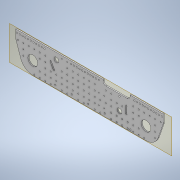
# Autodesk Inventor part: inside_plate
Saved by Autodesk Inventor 2022 (Build 260153000, 153)
## iProperties
Created: 2021-07-14
Part Number: inside_plate
Material: Generic
Document SubType Name: Modeling
Designer: gfellows
Density: 1 g/cm^3
Appearance: Default
Author: gfellows
Autodesk Inventor part; units mm, degrees
ref_plane "YZ Plane" through (0, 0, 0) normal (1, 0, 0) x (0, 1, 0)
ref_plane "XZ Plane" through (0, 0, 0) normal (0, 1, 0) x (-1, 0, 0)
ref_plane "XY Plane" through (0, 0, 0) normal (0, 0, 1) x (1, 0, 0)
ref_plane "Work Plane1" through (165.1, 7.35, 75.175) normal (0, 0, 1) x (1, 0, 0)
sketch "Sketch1" plane through (165.1, 7.35, 75.175) normal (0, 0, 1) x (1, 0, 0)
  circle A0 centre (165.1, -7.35) radius 14.2748 projected
  circle A1 centre (-165.1, -7.35) radius 14.2748 projected
  circle A2 centre (87.5579, -8.15) radius 7.008 projected
  circle A3 centre (-97.8958, 31.6508) radius 7.008 construction
  line L0 (59.5579, -27.1492) -> (-64.3191, -27.1492) construction
  line L1 (-64.3191, 10.8492) -> (59.5579, 10.8492) construction
  line L2 (-64.3191, -27.1492) -> (-64.3191, 10.8492) construction
  line L3 (59.5579, 10.8492) -> (59.5579, -27.1492) construction
  line L4 (73.4511, 1.35) -> (73.4511, -17.65) construction
  line L5 (59.5579, 1.35) -> (73.4511, 1.35) construction
  line L6 (73.4511, -17.65) -> (59.5579, -17.65) construction
  line L7 (113.5579, -44.65) -> (89.5579, -44.65) construction
  line L8 (89.5579, -44.65) -> (89.5579, -20.65) construction
  line L9 (85.5579, -20.65) -> (85.5579, -44.65) construction
  line L10 (85.5579, -44.65) -> (61.5579, -44.65) construction
  line L11 (61.5579, -44.65) -> (61.5579, -20.65) construction
  line L12 (61.5579, -20.65) -> (85.5579, -20.65) construction
  line L13 (89.5579, -20.65) -> (113.5579, -20.65) construction
  line L14 (113.5579, -20.65) -> (113.5579, -44.65) construction
  arc A4 (56.5579, -44.65) -> (60.5579, -40.65) centre (56.5579, -40.65) ccw construction
  arc A5 (-200.3988, -19.4033) -> (-165.1, -44.65) centre (-165.1, -7.35) ccw projected
  line L15 (215.1, 47.65) -> (-215.1, 47.65) projected
  arc A6 (165.1, -44.65) -> (200.3988, -19.4033) centre (165.1, -7.35) ccw projected
  arc A7 (114.5579, -40.65) -> (118.5579, -44.65) centre (118.5579, -40.65) ccw construction
  line L16 (114.5579, -23.65) -> (114.5579, -40.65) construction
  arc A8 (114.5579, -23.65) -> (110.5579, -19.65) centre (110.5579, -23.65) ccw construction
  line L17 (64.5579, -19.65) -> (110.5579, -19.65) construction
  arc A9 (64.5579, -19.65) -> (60.5579, -23.65) centre (64.5579, -23.65) ccw construction
  line L18 (60.5579, -40.65) -> (60.5579, -23.65) construction
  circle A10 centre (-165.1, -7.35) radius 14.2748 projected
  circle A11 centre (165.1, -7.35) radius 14.2748 projected
  circle A12 centre (-96.2421, 28.6508) radius 7.008 projected
  circle A13 centre (87.5579, -8.15) radius 7.008 projected
  line L19 (56.5579, -44.65) -> (118.5579, -44.65)
  circle A14 centre (63.5579, -24.65) radius 2
  circle A15 centre (79.5579, -24.65) radius 2
  circle A16 centre (63.5579, -40.65) radius 2
  circle A17 centre (79.5579, -40.65) radius 2
  circle A18 centre (95.5579, -24.65) radius 2
  circle A19 centre (111.5579, -24.65) radius 2
  circle A20 centre (111.5579, -40.65) radius 2
  circle A21 centre (95.5579, -40.65) radius 2
  circle A22 centre (27.1704, 7.85) radius 1.3526
  circle A23 centre (43.1704, 7.85) radius 1.3526
  circle A24 centre (27.1704, -24.15) radius 1.3526
  circle A25 centre (43.1704, -24.15) radius 1.3526
  line L20 (27.1704, 7.85) -> (43.1704, -24.15) construction
  line L21 (73.4511, -8.15) -> (-64.3191, -8.15) construction
  line L22 (-165.1, -44.65) -> (56.5579, -44.65) projected
  line L23 (-214.6708, 22.3931) -> (-200.3988, -19.4033) projected
  line L24 (-215.1, 47.65) -> (-215.1, 24.9782) projected
  line L25 (200.3988, -19.4033) -> (214.6708, 22.3931) projected
  line L26 (118.5579, -44.65) -> (165.1, -44.65) projected
  arc A26 (214.6708, 22.3931) -> (215.1, 24.9782) centre (207.1, 24.9782) ccw projected
  arc A27 (-215.1, 24.9782) -> (-214.6708, 22.3931) centre (-207.1, 24.9782) ccw projected
  circle A28 centre (-4.9, 39.65) radius 2 projected
  line L27 (31.1, 47.65) -> (31.1, 35.65) projected
  line L28 (-56.9, 47.65) -> (31.1, 47.65) projected
  line L29 (-56.9, 47.65) -> (-56.9, 35.65) projected
  line L30 (-56.9, 35.65) -> (31.1, 35.65) projected
  circle A29 centre (11.1, 39.65) radius 2 projected
  circle A30 centre (3.1, 39.65) radius 2 projected
  circle A31 centre (-4.9, 39.65) radius 2 projected
  circle A32 centre (-12.9, 39.65) radius 2 projected
  circle A33 centre (-20.9, 39.65) radius 2 projected
  circle A34 centre (-28.9, 39.65) radius 2 projected
  circle A35 centre (-36.9, 39.65) radius 2 projected
  circle A36 centre (-44.9, 39.65) radius 2 projected
  circle A37 centre (-52.9, 39.65) radius 2 projected
  circle A38 centre (19.1, 39.65) radius 2 projected
  circle A39 centre (27.1, 39.65) radius 2 projected
  line L31 (-215.1, 45.15) -> (-127.1, 45.15) projected
  line L32 (-127.1, 47.65) -> (-127.1, 35.65) projected
  line L33 (-215.1, 47.65) -> (-127.1, 47.65) projected
  line L34 (-215.1, 47.65) -> (-215.1, 35.65) projected
  line L35 (-215.1, 35.65) -> (-127.1, 35.65) projected
  circle A40 centre (-147.1, 39.65) radius 2 projected
  circle A41 centre (-155.1, 39.65) radius 2 projected
  circle A42 centre (-163.1, 39.65) radius 2 projected
  circle A43 centre (-171.1, 39.65) radius 2 projected
  circle A44 centre (-179.1, 39.65) radius 2 projected
  circle A45 centre (-187.1, 39.65) radius 2 projected
  circle A46 centre (-195.1, 39.65) radius 2 projected
  circle A47 centre (-203.1, 39.65) radius 2 projected
  circle A48 centre (-211.1, 39.65) radius 2 projected
  circle A49 centre (-139.1, 39.65) radius 2 projected
  circle A50 centre (-131.1, 39.65) radius 2 projected
  line L36 (215.1, 47.65) -> (215.1, 35.65) projected
  line L37 (127.1, 47.65) -> (215.1, 47.65) projected
  line L38 (127.1, 47.65) -> (127.1, 35.65) projected
  line L39 (127.1, 35.65) -> (215.1, 35.65) projected
  circle A51 centre (195.1, 39.65) radius 2 projected
  circle A52 centre (187.1, 39.65) radius 2 projected
  circle A53 centre (179.1, 39.65) radius 2 projected
  circle A54 centre (171.1, 39.65) radius 2 projected
  circle A55 centre (163.1, 39.65) radius 2 projected
  circle A56 centre (155.1, 39.65) radius 2 projected
  circle A57 centre (147.1, 39.65) radius 2 projected
  circle A58 centre (139.1, 39.65) radius 2 projected
  circle A59 centre (131.1, 39.65) radius 2 projected
  circle A60 centre (203.1, 39.65) radius 2 projected
  circle A61 centre (211.1, 39.65) radius 2 projected
  line L40 (215.1, 24.9782) -> (215.1, 47.65) projected
  arc A62 (109.4269, 14.5493) -> (105.4269, 14.5493) centre (107.4269, 14.5493) ccw projected
  line L41 (105.4269, -5.4507) -> (105.4269, 14.5493) projected
  arc A63 (105.4269, -5.4507) -> (109.4269, -5.4507) centre (107.4269, -5.4507) ccw projected
  line L42 (109.4269, 14.5493) -> (109.4269, -5.4507) projected
  arc A64 (-105.2208, -1.6588) -> (-101.6761, 0.1945) centre (-103.4484, -0.7322) ccw projected
  line L43 (-110.9425, 17.9183) -> (-101.6761, 0.1945) projected
  arc A65 (-110.9425, 17.9183) -> (-114.4873, 16.065) centre (-112.7149, 16.9916) ccw projected
  line L44 (-105.2208, -1.6588) -> (-114.4873, 16.065) projected
  circle A66 centre (-139.1, 39.65) radius 2 projected
  circle A67 centre (-155.1, 39.65) radius 2 projected
  circle A68 centre (-179.1, 39.65) radius 2 projected
  circle A69 centre (-187.1, 39.65) radius 2 projected
  circle A70 centre (-203.1, 39.65) radius 2 projected
  circle A71 centre (211.1, 39.65) radius 2 projected
  circle A72 centre (195.1, 39.65) radius 2 projected
  circle A73 centre (179.1, 39.65) radius 2 projected
  circle A74 centre (163.1, 39.65) radius 2 projected
  circle A75 centre (131.1, 39.65) radius 2 projected
  circle A76 centre (139.1, 39.65) radius 2 projected
  circle A77 centre (147.1, 39.65) radius 2 projected
  circle A78 centre (155.1, 39.65) radius 2 projected
  circle A79 centre (171.1, 39.65) radius 2 projected
  circle A80 centre (187.1, 39.65) radius 2 projected
  circle A81 centre (203.1, 39.65) radius 2 projected
  circle A82 centre (-211.1, 39.65) radius 2 projected
  circle A83 centre (-195.1, 39.65) radius 2 projected
  circle A84 centre (-171.1, 39.65) radius 2 projected
  circle A85 centre (-163.1, 39.65) radius 2 projected
  circle A86 centre (-147.1, 39.65) radius 2 projected
  circle A87 centre (-131.1, 39.65) radius 2 projected
  circle A88 centre (87.5579, 28.6508) radius 2 projected
  circle A89 centre (-99.4421, -35.8996) radius 2 projected
  circle A90 centre (-51.4421, -35.8996) radius 2 projected
  circle A91 centre (-3.4421, -35.8996) radius 2 projected
  circle A92 centre (44.5579, -35.8996) radius 2 projected
  circle A93 centre (119.5579, -39.65) radius 2 projected
  line L45 (63.5579, -24.65) -> (79.5579, -40.65) construction
  line L46 (95.5579, -24.65) -> (111.5579, -40.65) construction
  line L47 (63.5579, -40.65) -> (79.5579, -24.65) construction
  line L48 (95.5579, -40.65) -> (111.5579, -24.65) construction
  circle A94 centre (-96.2421, 28.6508) radius 6.25 construction
  circle A95 centre (-96.2421, 28.6508) radius 13.4851 projected
  circle A96 centre (-97.8958, 31.6508) radius 6.35 construction
  circle A97 centre (-96.2421, 28.6508) radius 7.0079
  circle A98 centre (52.9299, -33.2) radius 1.65 projected
  circle A99 centre (52.9299, 43) radius 1.65 projected
  circle A100 centre (-124.8701, -33.2) radius 1.65 projected
  circle A101 centre (-124.8701, 43) radius 1.65 projected
  point P0 (35.1704, -8.15)
  point P1 (207.1, 24.9782)
  point P2 (71.5579, -32.65)
  point P3 (103.5579, -32.65)
  dimension "d2" = 4
  dimension "d5" = 16
  dimension "d8" = 16
  dimension "d11" = 4
  dimension "d12" = 2
  dimension "d15" = 32
  dimension "d20" = 2.7051
  dimension "d23" = 16
  dimension "d30" = 31.9999
  dimension "d35" = 52.3875
  dimension "d36" = 32
  dimension "d37" = 12.7
  dimension "d38" = 14.0157
  constraints: 14 centre point, 14 end point, 5 midpoint, 4 horizontal, 2 coincident, 2 vertical, 1 point on line, 1 tangent, 20 other
  measures "d2" diameter of A14
  measures "d5" distance of L45.start L47.end
  measures "d8" distance of L45.start L47.start
  measures "d11" distance from line of L12 L45.start
  measures "d12" distance from line of L11 L45.start
  measures "d15" distance of L45.start L46.start
  measures "d20" diameter of A22
  measures "d23" distance of L20.start A23.centre
  measures "d30" distance of L20.start A24.centre
  measures "d35" distance of A2.centre point (35.17, -8.15)
  measures "d36" distance of point (103.558, -32.65) point (71.558, -32.65)
  measures "d37" diameter of A96
  measures "d38" diameter of A97
extrude "Extrusion1" add sketch "Sketch1" along normal blind 3.175 contours L23 A27 L24 L35 L32 L15 L29 L30 L27 L38 L39 L40 A26 L25 A6 L26 L19 L22 A5 | L24 L31 L32 L35 | L24 L15 L32 L31 | L15 L27 L30 L29 | L39 L38 L15 L36 | A95 | A98 | A99 | A100 | A101
sketch "Sketch2" plane through (165.1, 7.35, 78.35) normal (0, 0, 1) x (1, 0, 0)
  circle A0 centre (63.5579, -24.65) radius 2 projected
  circle A1 centre (79.5579, -24.65) radius 2 projected
  circle A2 centre (79.5579, -40.65) radius 2 projected
  circle A3 centre (63.5579, -40.65) radius 2 projected
  line L0 (215.1, 24.9782) -> (215.1, 47.65) projected
  line L1 (215.1, 47.65) -> (-215.1, 47.65) projected
  line L2 (-215.1, 47.65) -> (-215.1, 24.9782) projected
  arc A4 (-215.1, 24.9782) -> (-214.6708, 22.3931) centre (-207.1, 24.9782) ccw projected
  line L3 (-214.6708, 22.3931) -> (-200.3988, -19.4033) projected
  arc A5 (-200.3988, -19.4033) -> (-165.1, -44.65) centre (-165.1, -7.35) ccw projected
  line L4 (-165.1, -44.65) -> (165.1, -44.65) projected
  arc A6 (165.1, -44.65) -> (200.3988, -19.4033) centre (165.1, -7.35) ccw projected
  line L5 (200.3988, -19.4033) -> (214.6708, 22.3931) projected
  arc A7 (214.6708, 22.3931) -> (215.1, 24.9782) centre (207.1, 24.9782) ccw projected
  circle A8 centre (-131.1, 39.65) radius 2 projected
  circle A9 centre (-211.1, 39.65) radius 2 projected
  circle A10 centre (-147.1, 39.65) radius 2 projected
  circle A11 centre (-155.1, 39.65) radius 2 projected
  circle A12 centre (-163.1, 39.65) radius 2 projected
  circle A13 centre (-171.1, 39.65) radius 2 projected
  circle A14 centre (-179.1, 39.65) radius 2 projected
  circle A15 centre (-187.1, 39.65) radius 2 projected
  circle A16 centre (-195.1, 39.65) radius 2 projected
  circle A17 centre (-203.1, 39.65) radius 2 projected
  circle A18 centre (-139.1, 39.65) radius 2 projected
  circle A19 centre (211.1, 39.65) radius 2 projected
  circle A20 centre (131.1, 39.65) radius 2 projected
  circle A21 centre (195.1, 39.65) radius 2 projected
  circle A22 centre (187.1, 39.65) radius 2 projected
  circle A23 centre (179.1, 39.65) radius 2 projected
  circle A24 centre (171.1, 39.65) radius 2 projected
  circle A25 centre (163.1, 39.65) radius 2 projected
  circle A26 centre (155.1, 39.65) radius 2 projected
  circle A27 centre (147.1, 39.65) radius 2 projected
  circle A28 centre (139.1, 39.65) radius 2 projected
  circle A29 centre (203.1, 39.65) radius 2 projected
  circle A30 centre (27.1, 39.65) radius 2 projected
  circle A31 centre (-52.9, 39.65) radius 2 projected
  circle A32 centre (-36.9, 39.65) radius 2 projected
  circle A33 centre (-20.9, 39.65) radius 2 projected
  circle A34 centre (3.1, 39.65) radius 2 projected
  circle A35 centre (-4.9, 39.65) radius 2 projected
  circle A36 centre (11.1, 39.65) radius 2 projected
  circle A37 centre (-12.9, 39.65) radius 2 projected
  circle A38 centre (-28.9, 39.65) radius 2 projected
  circle A39 centre (-44.9, 39.65) radius 2 projected
  circle A40 centre (19.1, 39.65) radius 2 projected
  circle A41 centre (-96.2421, 28.6508) radius 7.0079 projected
  line L6 (105.4269, -5.4507) -> (105.4269, 14.5493) projected
  arc A42 (109.4269, 14.5493) -> (105.4269, 14.5493) centre (107.4269, 14.5493) ccw projected
  line L7 (109.4269, 14.5493) -> (109.4269, -5.4507) projected
  arc A43 (105.4269, -5.4507) -> (109.4269, -5.4507) centre (107.4269, -5.4507) ccw projected
  line L8 (-110.9425, 17.9183) -> (-101.6761, 0.1945) projected
  arc A44 (-105.2208, -1.6588) -> (-101.6761, 0.1945) centre (-103.4484, -0.7322) ccw projected
  line L9 (-105.2208, -1.6588) -> (-114.4873, 16.065) projected
  arc A45 (-110.9425, 17.9183) -> (-114.4873, 16.065) centre (-112.7149, 16.9916) ccw projected
  circle A46 centre (44.5579, -35.8996) radius 2 projected
  circle A47 centre (-51.4421, -35.8996) radius 2 projected
  circle A48 centre (87.5579, 28.6508) radius 2 projected
  circle A49 centre (27.1704, -24.15) radius 1.3526 projected
  circle A50 centre (27.1704, 7.85) radius 1.3526 projected
  circle A51 centre (111.5579, -40.65) radius 2 projected
  circle A52 centre (95.5579, -24.65) radius 2 projected
  circle A53 centre (165.1, -7.35) radius 14.2748 projected
  circle A54 centre (-165.1, -7.35) radius 14.2748 projected
  circle A55 centre (87.5579, -8.15) radius 7.008 projected
  circle A56 centre (63.5579, -24.65) radius 2 projected
  circle A57 centre (79.5579, -24.65) radius 2 projected
  circle A58 centre (63.5579, -40.65) radius 2 projected
  circle A59 centre (79.5579, -40.65) radius 2 projected
  circle A60 centre (111.5579, -24.65) radius 2 projected
  circle A61 centre (95.5579, -40.65) radius 2 projected
  circle A62 centre (43.1704, 7.85) radius 1.3526 projected
  circle A63 centre (43.1704, -24.15) radius 1.3526 projected
  circle A64 centre (-99.4421, -35.8996) radius 2 projected
  circle A65 centre (-3.4421, -35.8996) radius 2 projected
  circle A66 centre (119.5579, -39.65) radius 2 projected
  circle A67 centre (-203.1, 39.65) radius 1.65
  circle A68 centre (111.5579, -40.65) radius 2 projected
  circle A69 centre (111.5579, -40.65) radius 1.65
  circle A70 centre (95.5579, -40.65) radius 1.65
  circle A71 centre (79.5579, -40.65) radius 1.65
  circle A72 centre (63.5579, -40.65) radius 1.65
  circle A73 centre (47.5579, -40.65) radius 1.65
  circle A74 centre (31.5579, -40.65) radius 1.65
  circle A75 centre (15.5579, -40.65) radius 1.65
  circle A76 centre (-0.4421, -40.65) radius 1.65
  circle A77 centre (-16.4421, -40.65) radius 1.65
  circle A78 centre (-32.4421, -40.65) radius 1.65
  circle A79 centre (-48.4421, -40.65) radius 1.65
  circle A80 centre (-64.4421, -40.65) radius 1.65
  circle A81 centre (-80.4421, -40.65) radius 1.65
  circle A82 centre (-96.4421, -40.65) radius 1.65
  circle A83 centre (-112.4421, -40.65) radius 1.65
  circle A84 centre (-128.4421, -40.65) radius 1.65
  circle A85 centre (-144.4421, -40.65) radius 1.65
  circle A86 centre (-160.4421, -40.65) radius 1.65
  circle A87 centre (-176.4421, -40.65) radius 1.65
  circle A88 centre (-192.4421, -40.65) radius 1.65
  circle A89 centre (-208.4421, -40.65) radius 1.65
  circle A90 centre (111.5579, -24.65) radius 1.65
  circle A91 centre (95.5579, -24.65) radius 1.65
  circle A92 centre (79.5579, -24.65) radius 1.65
  circle A93 centre (63.5579, -24.65) radius 1.65
  circle A94 centre (47.5579, -24.65) radius 1.65
  circle A95 centre (31.5579, -24.65) radius 1.65
  circle A96 centre (15.5579, -24.65) radius 1.65
  circle A97 centre (-0.4421, -24.65) radius 1.65
  circle A98 centre (-16.4421, -24.65) radius 1.65
  circle A99 centre (-32.4421, -24.65) radius 1.65
  circle A100 centre (-48.4421, -24.65) radius 1.65
  circle A101 centre (-64.4421, -24.65) radius 1.65
  circle A102 centre (-80.4421, -24.65) radius 1.65
  circle A103 centre (-96.4421, -24.65) radius 1.65
  circle A104 centre (-112.4421, -24.65) radius 1.65
  circle A105 centre (-128.4421, -24.65) radius 1.65
  circle A106 centre (-144.4421, -24.65) radius 1.65
  circle A107 centre (-160.4421, -24.65) radius 1.65
  circle A108 centre (-176.4421, -24.65) radius 1.65
  circle A109 centre (-192.4421, -24.65) radius 1.65
  circle A110 centre (-208.4421, -24.65) radius 1.65
  circle A111 centre (111.5579, -8.65) radius 1.65
  circle A112 centre (95.5579, -8.65) radius 1.65
  circle A113 centre (79.5579, -8.65) radius 1.65
  circle A114 centre (63.5579, -8.65) radius 1.65
  circle A115 centre (47.5579, -8.65) radius 1.65
  circle A116 centre (31.5579, -8.65) radius 1.65
  circle A117 centre (15.5579, -8.65) radius 1.65
  circle A118 centre (-0.4421, -8.65) radius 1.65
  circle A119 centre (-16.4421, -8.65) radius 1.65
  circle A120 centre (-32.4421, -8.65) radius 1.65
  circle A121 centre (-48.4421, -8.65) radius 1.65
  circle A122 centre (-64.4421, -8.65) radius 1.65
  circle A123 centre (-80.4421, -8.65) radius 1.65
  circle A124 centre (-96.4421, -8.65) radius 1.65
  circle A125 centre (-112.4421, -8.65) radius 1.65
  circle A126 centre (-128.4421, -8.65) radius 1.65
  circle A127 centre (-144.4421, -8.65) radius 1.65
  circle A128 centre (-160.4421, -8.65) radius 1.65
  circle A129 centre (-176.4421, -8.65) radius 1.65
  circle A130 centre (-192.4421, -8.65) radius 1.65
  circle A131 centre (-208.4421, -8.65) radius 1.65
  circle A132 centre (111.5579, 7.35) radius 1.65
  circle A133 centre (95.5579, 7.35) radius 1.65
  circle A134 centre (79.5579, 7.35) radius 1.65
  circle A135 centre (63.5579, 7.35) radius 1.65
  circle A136 centre (47.5579, 7.35) radius 1.65
  circle A137 centre (31.5579, 7.35) radius 1.65
  circle A138 centre (15.5579, 7.35) radius 1.65
  circle A139 centre (-0.4421, 7.35) radius 1.65
  circle A140 centre (-16.4421, 7.35) radius 1.65
  circle A141 centre (-32.4421, 7.35) radius 1.65
  circle A142 centre (-48.4421, 7.35) radius 1.65
  circle A143 centre (-64.4421, 7.35) radius 1.65
  circle A144 centre (-80.4421, 7.35) radius 1.65
  circle A145 centre (-96.4421, 7.35) radius 1.65
  circle A146 centre (-112.4421, 7.35) radius 1.65
  circle A147 centre (-128.4421, 7.35) radius 1.65
  circle A148 centre (-144.4421, 7.35) radius 1.65
  circle A149 centre (-160.4421, 7.35) radius 1.65
  circle A150 centre (-176.4421, 7.35) radius 1.65
  circle A151 centre (-192.4421, 7.35) radius 1.65
  circle A152 centre (-208.4421, 7.35) radius 1.65
  circle A153 centre (111.5579, 23.35) radius 1.65
  circle A154 centre (95.5579, 23.35) radius 1.65
  circle A155 centre (79.5579, 23.35) radius 1.65
  circle A156 centre (63.5579, 23.35) radius 1.65
  circle A157 centre (47.5579, 23.35) radius 1.65
  circle A158 centre (31.5579, 23.35) radius 1.65
  circle A159 centre (15.5579, 23.35) radius 1.65
  circle A160 centre (-0.4421, 23.35) radius 1.65
  circle A161 centre (-16.4421, 23.35) radius 1.65
  circle A162 centre (-32.4421, 23.35) radius 1.65
  circle A163 centre (-48.4421, 23.35) radius 1.65
  circle A164 centre (-64.4421, 23.35) radius 1.65
  circle A165 centre (-80.4421, 23.35) radius 1.65
  circle A166 centre (-96.4421, 23.35) radius 1.65
  circle A167 centre (-112.4421, 23.35) radius 1.65
  circle A168 centre (-128.4421, 23.35) radius 1.65
  circle A169 centre (-144.4421, 23.35) radius 1.65
  circle A170 centre (-160.4421, 23.35) radius 1.65
  circle A171 centre (-176.4421, 23.35) radius 1.65
  circle A172 centre (-192.4421, 23.35) radius 1.65
  circle A173 centre (-208.4421, 23.35) radius 1.65
  circle A174 centre (111.5579, 39.35) radius 1.65
  circle A175 centre (95.5579, 39.35) radius 1.65
  circle A176 centre (79.5579, 39.35) radius 1.65
  circle A177 centre (63.5579, 39.35) radius 1.65
  circle A178 centre (47.5579, 39.35) radius 1.65
  circle A179 centre (31.5579, 39.35) radius 1.65
  circle A180 centre (15.5579, 39.35) radius 1.65
  circle A181 centre (-0.4421, 39.35) radius 1.65
  circle A182 centre (-16.4421, 39.35) radius 1.65
  circle A183 centre (-32.4421, 39.35) radius 1.65
  circle A184 centre (-48.4421, 39.35) radius 1.65
  circle A185 centre (-64.4421, 39.35) radius 1.65
  circle A186 centre (-80.4421, 39.35) radius 1.65
  circle A187 centre (-96.4421, 39.35) radius 1.65
  circle A188 centre (-112.4421, 39.35) radius 1.65
  circle A189 centre (-128.4421, 39.35) radius 1.65
  circle A190 centre (-144.4421, 39.35) radius 1.65
  circle A191 centre (-160.4421, 39.35) radius 1.65
  circle A192 centre (-176.4421, 39.35) radius 1.65
  circle A193 centre (-192.4421, 39.35) radius 1.65
  circle A194 centre (-208.4421, 39.35) radius 1.65
  circle A195 centre (127.5579, -40.65) radius 1.65
  circle A196 centre (143.5579, -40.65) radius 1.65
  circle A197 centre (159.5579, -40.65) radius 1.65
  circle A198 centre (175.5579, -40.65) radius 1.65
  circle A199 centre (191.5579, -40.65) radius 1.65
  circle A200 centre (207.5579, -40.65) radius 1.65
  circle A201 centre (111.5579, -24.65) radius 1.65
  circle A202 centre (127.5579, -24.65) radius 1.65
  circle A203 centre (143.5579, -24.65) radius 1.65
  circle A204 centre (159.5579, -24.65) radius 1.65
  circle A205 centre (175.5579, -24.65) radius 1.65
  circle A206 centre (191.5579, -24.65) radius 1.65
  circle A207 centre (207.5579, -24.65) radius 1.65
  circle A208 centre (111.5579, -8.65) radius 1.65
  circle A209 centre (127.5579, -8.65) radius 1.65
  circle A210 centre (143.5579, -8.65) radius 1.65
  circle A211 centre (159.5579, -8.65) radius 1.65
  circle A212 centre (175.5579, -8.65) radius 1.65
  circle A213 centre (191.5579, -8.65) radius 1.65
  circle A214 centre (207.5579, -8.65) radius 1.65
  circle A215 centre (111.5579, 7.35) radius 1.65
  circle A216 centre (127.5579, 7.35) radius 1.65
  circle A217 centre (143.5579, 7.35) radius 1.65
  circle A218 centre (159.5579, 7.35) radius 1.65
  circle A219 centre (175.5579, 7.35) radius 1.65
  circle A220 centre (191.5579, 7.35) radius 1.65
  circle A221 centre (207.5579, 7.35) radius 1.65
  circle A222 centre (111.5579, 23.35) radius 1.65
  circle A223 centre (127.5579, 23.35) radius 1.65
  circle A224 centre (143.5579, 23.35) radius 1.65
  circle A225 centre (159.5579, 23.35) radius 1.65
  circle A226 centre (175.5579, 23.35) radius 1.65
  circle A227 centre (191.5579, 23.35) radius 1.65
  circle A228 centre (207.5579, 23.35) radius 1.65
  circle A229 centre (111.5579, 39.35) radius 1.65
  circle A230 centre (127.5579, 39.35) radius 1.65
  circle A231 centre (143.5579, 39.35) radius 1.65
  circle A232 centre (159.5579, 39.35) radius 1.65
  circle A233 centre (175.5579, 39.35) radius 1.65
  circle A234 centre (191.5579, 39.35) radius 1.65
  circle A235 centre (207.5579, 39.35) radius 1.65
  dimension "d39" = 3.3
  dimension "d40" = 3.3
  dimension "d43" = 16
  dimension "d46" = 16
  dimension "d51" = 16
  dimension "d54" = 16
  constraints: 168 centre point, 2 coincident, 2 horizontal, 2 vertical, 332 other
  measures "d39" diameter of A67
  measures "d40" diameter of A69
  measures "d43" distance of A69.centre A70.centre
  measures "d46" distance of A69.centre A90.centre
  measures "d51" distance of A69.centre A195.centre
  measures "d54" distance of A69.centre A201.centre
extrude "Extrusion2" cut sketch "Sketch2" against normal through all contours A74 | A75 | A77 | A78 | A80 | A81 | A83 | A84 | A85 | A86 | A96 | A97 | A98 | A99 | A100 | A101 | A102 | A103 | A104 | A105 | A106 | A114 | A115 | A116 | A117 | A118 | A119 | A120 | A121 | A122 | A123 | A124 | A125 | A126 | A130 | A133 | A134 | A135 | A138 | A139 | A140 | A141 | A142 | A143 | A144 | A147 | A148 | A151 | A156 | A157 | A159 | A160 | A161 | A162 | A163 | A164 | A168 | A169 | A170 | A171 | A172 | A173 | A174 | A175 | A176 | A177 | A178 | A185 | A186 | A195 | A196 | A197 | A202 | A203 | A206 | A209 | A213 | A216 | A217 | A220 | A223 | A224 | A225 | A226 | A227 | A228
sketch "Sketch3" plane through (165.1, 7.35, 78.35) normal (0, 0, 1) x (1, 0, 0)
  circle A0 centre (-96.4421, -8.65) radius 1.65 projected
  circle A1 centre (127.5579, -24.65) radius 1.65 projected
  circle A2 centre (-16.4421, -40.65) radius 1.65 projected
  circle A3 centre (-0.4421, -24.65) radius 1.65 projected
  circle A4 centre (-48.4421, -8.65) radius 1.65 projected
  circle A5 centre (-16.4421, -8.65) radius 1.65 projected
  circle A6 centre (-16.4421, 23.35) radius 1.65 projected
  circle A7 centre (-176.4421, 23.35) radius 1.65 projected
  circle A8 centre (-128.4421, 7.35) radius 1.65 projected
  circle A9 centre (-144.4421, -24.65) radius 1.65 projected
  circle A10 centre (-112.4421, -40.65) radius 1.65 projected
  circle A11 centre (-80.4421, -24.65) radius 1.65 projected
  circle A12 centre (-64.4421, -24.65) radius 1.65 projected
  circle A13 centre (-80.4421, 39.35) radius 1.65 projected
  circle A14 centre (15.5579, -8.65) radius 1.65 projected
  circle A15 centre (63.5579, -8.65) radius 1.65 projected
  circle A16 centre (-64.4421, -40.65) radius 1.65 projected
  circle A17 centre (175.5579, 23.35) radius 1.65 projected
  circle A18 centre (111.5579, 39.35) radius 1.65 projected
  circle A19 centre (47.5579, 39.35) radius 1.65 projected
  circle A20 centre (127.5579, 7.35) radius 1.65 projected
  circle A21 centre (159.5579, -40.65) radius 1.65 projected
  circle A22 centre (127.5579, -8.65) radius 1.65 projected
  circle A23 centre (63.5579, 39.35) radius 1.65 projected
  circle A24 centre (127.5579, 23.35) radius 1.65 projected
  circle A25 centre (191.5579, 7.35) radius 1.65 projected
  circle A26 centre (31.5579, -40.65) radius 1.65 projected
  circle A27 centre (63.5579, 7.35) radius 1.65 projected
  circle A28 centre (15.5579, 7.35) radius 1.65 projected
  circle A29 centre (-80.4421, 7.35) radius 1.65 projected
  circle A30 centre (-64.4421, -8.65) radius 1.65 projected
  circle A31 centre (-208.4421, 23.35) radius 1.65 projected
  circle A32 centre (-128.4421, -40.65) radius 1.65 projected
  circle A33 centre (-112.4421, -24.65) radius 1.65 projected
  circle A34 centre (-128.4421, 23.35) radius 1.65 projected
  circle A35 centre (-192.4421, 23.35) radius 1.65 projected
  circle A36 centre (-0.4421, 23.35) radius 1.65 projected
  circle A37 centre (-16.4421, 7.35) radius 1.65 projected
  circle A38 centre (-32.4421, 7.35) radius 1.65 projected
  circle A39 centre (-16.4421, -24.65) radius 1.65 projected
  circle A40 centre (143.5579, -24.65) radius 1.65 projected
  circle A41 centre (143.5579, 7.35) radius 1.65 projected
  circle A42 centre (207.5579, 23.35) radius 1.65 projected
  circle A43 centre (-112.4421, -8.65) radius 1.65 projected
  circle A44 centre (127.5579, -40.65) radius 1.65 projected
  circle A45 centre (-32.4421, -40.65) radius 1.65 projected
  circle A46 centre (15.5579, -24.65) radius 1.65 projected
  circle A47 centre (-32.4421, -8.65) radius 1.65 projected
  circle A48 centre (-0.4421, 7.35) radius 1.65 projected
  circle A49 centre (-32.4421, 23.35) radius 1.65 projected
  circle A50 centre (-160.4421, 23.35) radius 1.65 projected
  circle A51 centre (-128.4421, -8.65) radius 1.65 projected
  circle A52 centre (-144.4421, -40.65) radius 1.65 projected
  circle A53 centre (-192.4421, 7.35) radius 1.65 projected
  circle A54 centre (-96.4421, -24.65) radius 1.65 projected
  circle A55 centre (-64.4421, 7.35) radius 1.65 projected
  circle A56 centre (-64.4421, 39.35) radius 1.65 projected
  circle A57 centre (47.5579, 23.35) radius 1.65 projected
  circle A58 centre (79.5579, 7.35) radius 1.65 projected
  circle A59 centre (-80.4421, -40.65) radius 1.65 projected
  circle A60 centre (159.5579, 23.35) radius 1.65 projected
  circle A61 centre (95.5579, 39.35) radius 1.65 projected
  circle A62 centre (47.5579, -8.65) radius 1.65 projected
  circle A63 centre (191.5579, -24.65) radius 1.65 projected
  circle A64 centre (191.5579, -8.65) radius 1.65 projected
  circle A65 centre (31.5579, -8.65) radius 1.65 projected
  circle A66 centre (79.5579, 39.35) radius 1.65 projected
  circle A67 centre (143.5579, 23.35) radius 1.65 projected
  circle A68 centre (191.5579, 23.35) radius 1.65 projected
  circle A69 centre (95.5579, 7.35) radius 1.65 projected
  circle A70 centre (63.5579, 23.35) radius 1.65 projected
  circle A71 centre (15.5579, 23.35) radius 1.65 projected
  circle A72 centre (-64.4421, 23.35) radius 1.65 projected
  circle A73 centre (-80.4421, -8.65) radius 1.65 projected
  circle A74 centre (-192.4421, -8.65) radius 1.65 projected
  circle A75 centre (-160.4421, -40.65) radius 1.65 projected
  circle A76 centre (-128.4421, -24.65) radius 1.65 projected
  circle A77 centre (-144.4421, 23.35) radius 1.65 projected
  circle A78 centre (-48.4421, 23.35) radius 1.65 projected
  circle A79 centre (-0.4421, -8.65) radius 1.65 projected
  circle A80 centre (-48.4421, 7.35) radius 1.65 projected
  circle A81 centre (15.5579, -40.65) radius 1.65 projected
  circle A82 centre (-32.4421, -24.65) radius 1.65 projected
  circle A83 centre (143.5579, -40.65) radius 1.65 projected
  circle A84 centre (-144.4421, 7.35) radius 1.65 projected
  circle A85 centre (-48.4421, -24.65) radius 1.65 projected
  line L0 (215.1, 24.9782) -> (215.1, 47.65) projected
  line L1 (215.1, 47.65) -> (-215.1, 47.65) projected
  line L2 (-215.1, 47.65) -> (-215.1, 24.9782) projected
  arc A86 (-215.1, 24.9782) -> (-214.6708, 22.3931) centre (-207.1, 24.9782) ccw projected
  line L3 (-214.6708, 22.3931) -> (-200.3988, -19.4033) projected
  arc A87 (-200.3988, -19.4033) -> (-165.1, -44.65) centre (-165.1, -7.35) ccw projected
  line L4 (-165.1, -44.65) -> (165.1, -44.65) projected
  arc A88 (165.1, -44.65) -> (200.3988, -19.4033) centre (165.1, -7.35) ccw projected
  line L5 (200.3988, -19.4033) -> (214.6708, 22.3931) projected
  arc A89 (214.6708, 22.3931) -> (215.1, 24.9782) centre (207.1, 24.9782) ccw projected
  circle A90 centre (-131.1, 39.65) radius 2 projected
  circle A91 centre (-211.1, 39.65) radius 2 projected
  circle A92 centre (-147.1, 39.65) radius 2 projected
  circle A93 centre (-155.1, 39.65) radius 2 projected
  circle A94 centre (-163.1, 39.65) radius 2 projected
  circle A95 centre (-171.1, 39.65) radius 2 projected
  circle A96 centre (-179.1, 39.65) radius 2 projected
  circle A97 centre (-187.1, 39.65) radius 2 projected
  circle A98 centre (-195.1, 39.65) radius 2 projected
  circle A99 centre (-203.1, 39.65) radius 2 projected
  circle A100 centre (-139.1, 39.65) radius 2 projected
  circle A101 centre (211.1, 39.65) radius 2 projected
  circle A102 centre (131.1, 39.65) radius 2 projected
  circle A103 centre (195.1, 39.65) radius 2 projected
  circle A104 centre (187.1, 39.65) radius 2 projected
  circle A105 centre (179.1, 39.65) radius 2 projected
  circle A106 centre (171.1, 39.65) radius 2 projected
  circle A107 centre (163.1, 39.65) radius 2 projected
  circle A108 centre (155.1, 39.65) radius 2 projected
  circle A109 centre (147.1, 39.65) radius 2 projected
  circle A110 centre (139.1, 39.65) radius 2 projected
  circle A111 centre (203.1, 39.65) radius 2 projected
  circle A112 centre (27.1, 39.65) radius 2 projected
  circle A113 centre (-52.9, 39.65) radius 2 projected
  circle A114 centre (-36.9, 39.65) radius 2 projected
  circle A115 centre (-20.9, 39.65) radius 2 projected
  circle A116 centre (3.1, 39.65) radius 2 projected
  circle A117 centre (-4.9, 39.65) radius 2 projected
  circle A118 centre (11.1, 39.65) radius 2 projected
  circle A119 centre (-12.9, 39.65) radius 2 projected
  circle A120 centre (-28.9, 39.65) radius 2 projected
  circle A121 centre (-44.9, 39.65) radius 2 projected
  circle A122 centre (19.1, 39.65) radius 2 projected
  circle A123 centre (-96.2421, 28.6508) radius 7.0079 projected
  line L6 (105.4269, -5.4507) -> (105.4269, 14.5493) projected
  arc A124 (109.4269, 14.5493) -> (105.4269, 14.5493) centre (107.4269, 14.5493) ccw projected
  line L7 (109.4269, 14.5493) -> (109.4269, -5.4507) projected
  arc A125 (105.4269, -5.4507) -> (109.4269, -5.4507) centre (107.4269, -5.4507) ccw projected
  line L8 (-110.9425, 17.9183) -> (-101.6761, 0.1945) projected
  arc A126 (-105.2208, -1.6588) -> (-101.6761, 0.1945) centre (-103.4484, -0.7322) ccw projected
  line L9 (-105.2208, -1.6588) -> (-114.4873, 16.065) projected
  arc A127 (-110.9425, 17.9183) -> (-114.4873, 16.065) centre (-112.7149, 16.9916) ccw projected
  circle A128 centre (44.5579, -35.8996) radius 2 projected
  circle A129 centre (-51.4421, -35.8996) radius 2 projected
  circle A130 centre (87.5579, 28.6508) radius 2 projected
  circle A131 centre (27.1704, -24.15) radius 1.3526 projected
  circle A132 centre (27.1704, 7.85) radius 1.3526 projected
  circle A133 centre (111.5579, -40.65) radius 2 projected
  circle A134 centre (95.5579, -24.65) radius 2 projected
  circle A135 centre (165.1, -7.35) radius 14.2748 projected
  circle A136 centre (-165.1, -7.35) radius 14.2748 projected
  circle A137 centre (87.5579, -8.15) radius 7.008 projected
  circle A138 centre (63.5579, -24.65) radius 2 projected
  circle A139 centre (79.5579, -24.65) radius 2 projected
  circle A140 centre (63.5579, -40.65) radius 2 projected
  circle A141 centre (79.5579, -40.65) radius 2 projected
  circle A142 centre (111.5579, -24.65) radius 2 projected
  circle A143 centre (95.5579, -40.65) radius 2 projected
  circle A144 centre (43.1704, 7.85) radius 1.3526 projected
  circle A145 centre (43.1704, -24.15) radius 1.3526 projected
  circle A146 centre (-99.4421, -35.8996) radius 2 projected
  circle A147 centre (-3.4421, -35.8996) radius 2 projected
  circle A148 centre (119.5579, -39.65) radius 2 projected
  line L10 (215.1, 47.65) -> (-215.1, 47.65) projected
  line L11 (39.8, 47.65) -> (118.4, 47.65)
  line L12 (118.4, 47.65) -> (118.4, 35.0008)
  line L13 (118.4, 35.0008) -> (39.8, 35.0008)
  line L14 (39.8, 35.0008) -> (39.8, 47.65)
  dimension "d59" = 12.7
  dimension "d60" = 12.7
  dimension "d61" = 6.35
  constraints: 8 end point, 2 parallel, 1 horizontal, 1 perpendicular, 1 point on line
  measures "d59" distance from line of L14 A112.centre
  measures "d60" distance from line of A102.centre L12
  measures "d61" distance from line of L13 A130.centre
extrude "Extrusion3" cut sketch "Sketch3" against normal blind 25.4 contours A18 | A19 | A23 | A61 | A66 | L12 L13 L14 L1
fillet "Fillet1" radius 8 2 edges at (204.9, 42.3508, 76.7625) (283.5, 42.3508, 76.7625)
body "Solid1"
